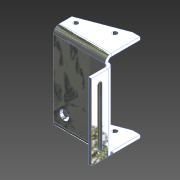
# Autodesk Inventor part: trackball_l
Saved by Autodesk Inventor 2018 (Build 220112000, 112)
## iProperties
Created: 2018-07-04
Part Number: trackball_l
Material: アルミニウム 6061
Document SubType Name: Sheet Metal
Designer: NaMACHAN
Mass: 19.4478 g
Surface Area: 80.3945 cm^2
Volume: 7.20289 cm^3
Density: 2.7 g/cm^3
Sheet Metal Rule: Default
Appearance: アルミニウム - フラット
Flat Pattern Width: 4.35239 cm
Flat Pattern Length: 9.70478 cm
Flat Pattern Area: 42.239 cm^2
Sheet Metal Width: 43.524 mm
Sheet Metal Length: 97.048 mm
Sheet Metal Area: 4223.898 mm^2
Author: NaMACHAN
Autodesk Inventor part; units mm, degrees
ref_plane "YZ Plane" through (0, 0, 0) normal (1, 0, 0) x (0, 1, 0)
ref_plane "XZ Plane" through (0, 0, 0) normal (0, 1, 0) x (-1, 0, 0)
ref_plane "XY Plane" through (0, 0, 0) normal (0, 0, 1) x (1, 0, 0)
sketch "スケッチ1" plane through (0, 0, 0) normal (0, 1, 0) x (-1, 0, 0)
  line L0 (-14, -27) -> (14, -27)
  line L1 (14, 27) -> (-14, 27)
  line L2 (-14, 27) -> (-14, -27)
  line L3 (-14, -27) -> (14, 27) construction
  line L4 (14, -27) -> (-14, 27) construction
  line L5 (14, -27) -> (14, 27)
  point P0 (0, 0)
  dimension "d0" = 28
  dimension "d1" = 54
  measures "d0" distance of L1.end L1.start
  measures "d1" distance of L1.start L0.end
extrude "プレート1" add sketch "スケッチ1" along normal blind 2
sketch "スケッチ2" plane through (-14, 0, 27) normal (0, 0, 1) x (1, 0, 0)
  line L0 (0, 2) -> (28, 2)
  line L1 (0, 2) -> (0, 12)
  line L2 (0, 12) -> (23, 23)
  line L3 (23, 23) -> (28, 23)
  line L4 (28, 23) -> (28, 2)
  line L5 (0, 0) -> (0, 2)
  line L6 (28, 2) -> (0, 2)
  point P0 (14, 0)
  dimension "d3" = 10
  dimension "d4" = 5
  dimension "d5" = 21
  measures "d3" distance of L0.start L1.end
  measures "d4" distance of L2.end L3.end
  measures "d5" distance between parallel lines of L3 L0
sheet face with bend "面2" sketch "スケッチ2" thickness 2 toward (0, 0, 1) bend radius 2
bend "曲げ1"
sketch "スケッチ3" plane through (14, 0, -27) normal (0, 0, -1) x (-1, 0, 0)
  line L0 (0, 0) -> (0, 2)
  line L1 (0, 2) -> (0, 23)
  line L2 (0, 23) -> (5, 23)
  line L3 (0, 23) -> (5, 23)
  line L4 (28, 12) -> (28, 4)
  line L5 (5, 23) -> (28, 12)
  line L6 (28, 0) -> (28, 2)
  line L7 (28, 12) -> (28, 2)
  line L8 (28, 2) -> (0, 2)
  point P0 (14, 0)
sheet face with bend "面3" sketch "スケッチ3" thickness 2 toward (0, 0, -1) bend radius 2
bend "曲げ2"
sketch "スケッチ4" plane through (14, 0, -29) normal (0, 0, -1) x (-1, 0, 0)
  line L0 (5, 23) -> (28, 12) projected
  line L1 (0, 23) -> (5, 23) projected
  line L2 (28, 4) -> (28, 12) projected
  point P0 (14, 0)
  point P1 (4.9573, 18.5865)
  point P2 (23, 9.9574)
  dimension "d16" = 4
  dimension "d17" = 4
  dimension "d18" = 20
  dimension "d44" = 5
  measures "d16" distance from line of L0 point (23, 9.957)
  measures "d17" distance from line of L0 point (4.957, 18.586)
  measures "d18" distance of point (4.957, 18.586) point (23, 9.957)
  measures "d44" distance from line of L2 point (23, 9.957)
hole "穴1" at (9.0427, 18.5865, -29) at (-9, 9.9574, -29) direction (0, 0, 1) diameter 3 end through all
sketch "スケッチ6" plane through (16, -2, -25) normal (1, 0, 0) x (0, -1, 0)
  line L0 (0, 50) -> (0, 0)
  line L1 (0, 0) -> (11, 0)
  line L2 (11, 0) -> (11, 50)
  line L3 (11, 50) -> (0, 50)
  constraints: 6 end point, 1 horizontal, 1 perpendicular, 1 vertical
edge flange "フランジ1" height 15 angle 90 thickness 2 bend radius 2 thickness toward (1, 0, 0) relief straight relief width 2 relief depth 1 edges at (14, 2, 0) wall of the first edge with corners at (16, -2, 25) (16, -2, -25) (16, -13, -25) (16, -13, 25)
bend "曲げ3"
corner "コーナー1"
sketch "スケッチ8" plane through (16, -13, -25) normal (-1, 0, 0) x (0, 0, 1)
  line L0 (44, 4) -> (6, 4)
  arc A0 (6, 7) -> (6, 4) centre (6, 5.5) ccw
  line L1 (6, 7) -> (44, 7)
  arc A1 (44, 4) -> (44, 7) centre (44, 5.5) ccw
  line L2 (50, 11) -> (50, 0) projected
  line L3 (0, 0) -> (0, 11) projected
  line L4 (50, 0) -> (0, 0) projected
  point P0 (25, 13)
  point P1 (50, 5.5)
  dimension "d66" = 6
  dimension "d67" = 6
  dimension "d69" = 1.5
  constraints: 4 end point, 4 point on circle, 4 tangent, 2 centre point, 1 horizontal, 1 horizontal alignment, 1 midpoint, 1 parallel
  measures "d66" distance from line of L2 A1.centre
  measures "d67" distance from line of L3 A0.centre
  measures "d69" radius of A1
extrude "押し出し2" cut sketch "スケッチ8" against normal blind 10
sketch "スケッチ9" plane through (0, 2, 0) normal (0, 1, 0) x (1, 0, 0)
  line L0 (14, 25) -> (-14, 25) projected
  line L1 (-14, -25) -> (-14, 25) projected
  point P0 (0, 0)
  point P1 (-7, 18)
  dimension "d72" = 7
  dimension "d73" = 7
  measures "d72" distance from line of L0 point (-7, 18)
  measures "d73" distance from line of L1 point (-7, 18)
hole "穴3" at (-7, 2, -18) direction (0, -1, 0) diameter 6 end through all
equation "\"d25\" = Thickness"
equation "\"d79\" = Thickness"
equation "\"d2\" = Thickness"
equation "\"d6\" = BendRadius"
equation "\"d7\" = BendReliefWidth"
equation "\"d9\" = MinimumRemnant"
equation "\"d8\" = BendReliefDepth"
equation "\"d10\" = TransitionRadius"
equation "\"d11\" = BendRadius"
equation "\"d12\" = BendReliefWidth"
equation "\"d14\" = MinimumRemnant"
equation "\"d13\" = BendReliefDepth"
equation "\"d15\" = TransitionRadius"
equation "\"d45\" = BendReliefWidth"
equation "\"d46\" = BendReliefDepth"
equation "\"d47\" = MinimumRemnant"
equation "\"d48\" = TransitionRadius"
equation "\"d51\" = BendRadius"
equation "\"d52\" = CornerReliefSize"
equation "\"d53\" = GapSize"
equation "\"d54\" = JacobiRadiusSize"
equation "\"BendRadius\" = Thickness"
equation "\"BendReliefWidth\" = Thickness"
equation "\"BendReliefDepth\" = 0.5 * Thickness"
equation "\"CornerReliefSize\" = 4 * Thickness"
equation "\"MinimumRemnant\" = 2 * Thickness"
equation "\"TransitionRadius\" = BendRadius"
equation "\"JacobiRadiusSize\" = Thickness"
equation "\"GapSize\" = Thickness"
equation "\"Thickness\" = 2"
